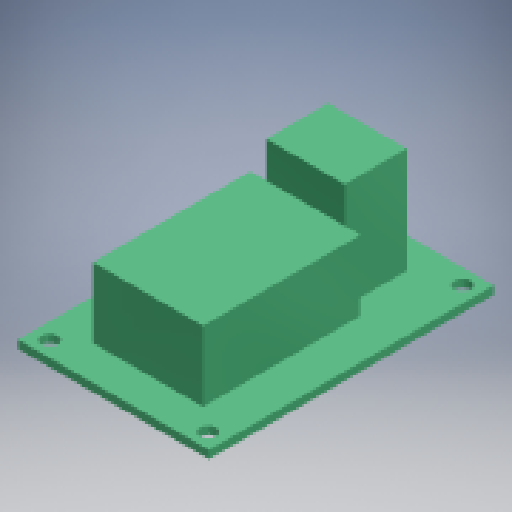
# Autodesk Inventor part: NAS_Splitter_PCB
Saved by Autodesk Inventor 2025.2 (Build 292293000, 293)
## iProperties
Created: 2025-02-16
Part Number: NAS_Splitter_PCB
Material: Generic
Document SubType Name: Modeling
Designer: Paul Linke
Density: 1 g/cm^3
Appearance: Green Polished
Author: Paul Linke
Autodesk Inventor part; units mm, degrees
ref_plane "YZ Plane" through (0, 0, 0) normal (1, 0, 0) x (0, 1, 0)
ref_plane "XZ Plane" through (0, 0, 0) normal (0, 1, 0) x (-1, 0, 0)
ref_plane "XY Plane" through (0, 0, 0) normal (0, 0, 1) x (1, 0, 0)
sketch "Sketch1" plane through (0, 0, 0) normal (0, 1, 0) x (-1, 0, 0)
  line L0 (92.3312, 46.4889) -> (54.1312, 46.4889)
  line L1 (54.1312, 46.4889) -> (54.1312, 103.4889)
  line L2 (54.1312, 103.4889) -> (92.3312, 103.4889)
  line L3 (92.3312, 103.4889) -> (92.3312, 46.4889)
  circle A0 centre (89.1312, 49.5389) radius 1.6
  circle A1 centre (57.3312, 49.5389) radius 1.6
  circle A2 centre (89.1312, 100.4389) radius 1.6
  circle A3 centre (57.3312, 100.4389) radius 1.6
  point P0 (0, 0)
  dimension "d0" = 57
  dimension "d1" = 38.2
  dimension "d2" = 3.2
  dimension "d3" = 3.2
  dimension "d4" = 3.05
  dimension "d11" = 3.05
  dimension "d12" = 3.2
  dimension "d13" = 3.05
  dimension "d14" = 3.05
  dimension "d15" = 3.2
  dimension "d16" = 3.2
  constraints: 8 end point, 4 centre point, 2 parallel, 1 horizontal, 1 perpendicular
  measures "d0" distance between parallel lines of L2 L0
  measures "d1" distance between parallel lines of L1 L3
  measures "d2" diameter of A0
  measures "d3" distance from line of L3 A0.centre
  measures "d4" distance from line of L0 A0.centre
  measures "d11" distance from line of L0 A1.centre
  measures "d12" distance from line of L1 A1.centre
  measures "d13" distance from line of L2 A3.centre
  measures "d14" distance from line of L2 A2.centre
  measures "d15" distance from line of L3 A2.centre
  measures "d16" distance from line of L1 A3.centre
extrude "Extrusion1" add sketch "Sketch1" along normal blind 1.6
sketch "Sketch2" plane through (0, 1.6, 0) normal (0, 1, 0) x (1, 0, 0)
  line L0 (-81.0812, -52.6889) -> (-65.3812, -52.6889)
  line L1 (-65.3812, -52.6889) -> (-65.3812, -65.0889)
  line L2 (-65.3812, -65.0889) -> (-81.0812, -65.0889)
  line L3 (-81.0812, -65.0889) -> (-81.0812, -52.6889)
  line L4 (-54.1312, -46.4889) -> (-92.3312, -46.4889) projected
  line L5 (-92.3312, -46.4889) -> (-92.3312, -103.4889) construction
  line L6 (-54.1312, -46.4889) -> (-92.3312, -103.4889) construction
  line L7 (-92.3312, -103.4889) -> (-54.1312, -103.4889) construction
  line L8 (-92.3312, -46.4889) -> (-54.1312, -103.4889) construction
  line L9 (-73.2312, -103.4889) -> (-73.2312, -46.4889) construction
  point P0 (0, 0)
  point P1 (-73.2312, -52.6889)
  dimension "d19" = 6.2
  dimension "d20" = 15.7
  dimension "d21" = 12.4
  constraints: 14 end point, 3 midpoint, 2 parallel, 1 horizontal, 1 perpendicular, 1 other
  measures "d19" distance between parallel lines of L0 L4
  measures "d20" distance between parallel lines of L1 L3
  measures "d21" distance from line of point (-73.231, -52.689) L2
extrude "Extrusion2" add sketch "Sketch2" along normal blind 21.2
sketch "Sketch3" plane through (0, 1.6, 0) normal (0, 1, 0) x (1, 0, 0)
  line L0 (-81.0812, -65.0889) -> (-65.3812, -65.0889) projected
  line L1 (-84.2537, -65.0889) -> (-62.2087, -65.0889)
  line L2 (-62.2087, -65.0889) -> (-62.2087, -96.5889)
  line L3 (-62.2087, -96.5889) -> (-84.2537, -96.5889)
  line L4 (-84.2537, -96.5889) -> (-84.2537, -65.0889)
  line L5 (-92.3312, -103.4889) -> (-54.1312, -103.4889) projected
  line L6 (-54.1312, -103.4889) -> (-54.1312, -46.4889) construction
  line L7 (-54.1312, -103.4889) -> (-92.3312, -46.4889) construction
  line L8 (-92.3312, -103.4889) -> (-54.1312, -46.4889) construction
  line L9 (-73.2312, -61.8477) -> (-73.2312, -121.9284) construction
  point P0 (0, 0)
  dimension "d24" = 6.9
  constraints: 14 end point, 2 parallel, 1 horizontal, 1 perpendicular, 1 vertical, 1 other
  measures "d24" distance between parallel lines of L5 L3
extrude "Extrusion3" add sketch "Sketch3" along normal blind 14
body "Solid1"
